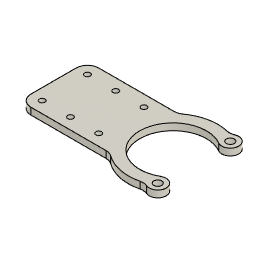
ZIMA-R_holder_flat (Autodesk Fusion 360 design; units mm, degrees)
Autodesk Fusion 360 part; units mm, degrees
sketch "Sketch1" plane through (0, 0, 0) normal (0, 0, 1) x (1, 0, 0)
  circle A0 centre (18.5, 32.0429) radius 7.5
  circle A1 centre (18.5, -32.0429) radius 7.5
  line L0 (0, 0) -> (80.5902, 0) construction
  line L1 (0, 0) -> (18.5, 32.0429) construction
  arc A2 (14.75, 25.5477) -> (14.75, -25.5477) centre (0, 0) ccw
  arc A3 (13.1121, 37.2602) -> (13.1121, -37.2602) centre (0, 0) ccw
  line L2 (-25.6953, 30) -> (-95.6953, 30)
  line L3 (-95.6953, -30) -> (-25.6953, -30)
  line L4 (0, 0) -> (-230.6084, 0) construction
  circle A4 centre (18.5, 32.0429) radius 3.5
  circle A5 centre (18.5, -32.0429) radius 3.5
  line L5 (-105.6953, 20) -> (-105.6953, -20)
  arc A6 (-95.6953, 30) -> (-105.6953, 20) centre (-95.6953, 20) ccw
  arc A7 (-105.6953, -20) -> (-95.6953, -30) centre (-95.6953, -20) ccw
  circle A8 centre (-95.6953, 20) radius 2.5
  circle A9 centre (-95.6953, -20) radius 2.5
  circle A10 centre (-45.6953, -20) radius 2.5
  circle A11 centre (-45.6953, 20) radius 2.5
  circle A12 centre (-70.6953, 20) radius 2.5
  circle A13 centre (-70.6953, -20) radius 2.5
  point P0 (-105.6953, 30)
  point P1 (-105.6953, -30)
  dimension "d1" = 59
  dimension "d2" = 10
  dimension "d3" = 60
  dimension "d4" = 15
  dimension "d5" = 60
  dimension "d23" = 7
  dimension "d25" = 80
  dimension "d26" = 10
  dimension "d27" = 5
  dimension "d28" = 5
  dimension "d29" = 50
  dimension "d30" = 25
  constraint coincident L0.start L1.start
  constraint tangent A0 A2
  constraint tangent A1 A2
  constraint horizontal L0
  constraint coincident A0.centre L1.end
  constraint symmetric A0.centre A1.centre L0
  constraint coincident A0 A2.start
  constraint coincident A1 A2.end
  constraint coincident A0 A3.start
  constraint coincident A1 A3.end
  constraint coincident A3 L2.start
  constraint coincident A3 L3.end
  constraint concentric A0 A4
  constraint concentric A1 A5
  constraint equal A4 A5
  constraint horizontal L2
  constraint symmetric L2 L3 L4
  constraint perpendicular L2 L5
  constraint perpendicular L3 L5
  constraint coincident P0 L2
  constraint coincident P0 L5
  constraint tangent L2 A6
  constraint tangent L5 A6
  constraint coincident P1 L3
  constraint coincident P1 L5
  constraint tangent L3 A7
  constraint tangent L5 A7
  constraint equal A6 A7
  constraint concentric A6 A8
  constraint concentric A7 A9
  constraint horizontal A6.centre A11.centre
  constraint symmetric L4 A10.centre A11.centre
  constraint equal A8 A11
  constraint equal A10 A11
  constraint equal A12 A13
  constraint equal A8 A12
  constraint symmetric L4 A12.centre A13.centre
  constraint horizontal A6.centre A12.centre
  measures "d1" diameter of A2
  measures "d2" distance of A2 A3
  measures "d3" angle of L0 L1
  measures "d4" diameter of A0
  measures "d5" distance of P0 P1
  measures "d23" diameter of A4
  measures "d25" distance of L2.start P0
  measures "d26" radius of A6
  measures "d27" diameter of A8
  measures "d28" diameter of A9
  measures "d29" distance of A6.centre A11.centre
  measures "d30" horizontal distance of A6.centre A12.centre
extrude "Extrude1" add sketch "Sketch1" along normal blind 6
fillet "Fillet1" radius 10 4 edges at (13.1121, 37.2602, 3) (-25.6953, 30, 3) (13.1121, -37.2602, 3) (-25.6953, -30, 3)
